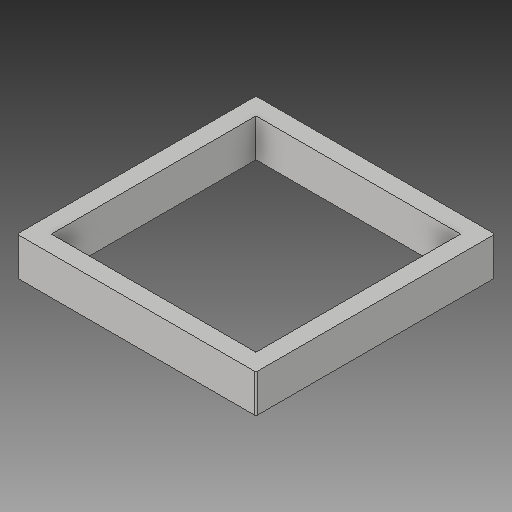
# Autodesk Inventor part: Bumpers
Saved by Autodesk Inventor 2019 (Build 230136000, 136)
## iProperties
Created: 2019-03-14
Part Number: Bumpers
Material: Generic
Document SubType Name: Modeling
Designer: josh
Density: 1 g/cm^3
Appearance: Default
Mass: 29193.8 g
Surface Area: 13341.7 cm^2
Volume: 29193.8 cm^3
Author: josh
Autodesk Inventor part; units mm, degrees
ref_plane "YZ Plane" through (0, 0, 0) normal (1, 0, 0) x (0, 1, 0)
ref_plane "XZ Plane" through (0, 0, 0) normal (0, 1, 0) x (-1, 0, 0)
ref_plane "XY Plane" through (0, 0, 0) normal (0, 0, 1) x (1, 0, 0)
sketch "Sketch5" plane through (0, 0, 0) normal (0, 1, 0) x (-1, 0, 0)
  line L0 (0, 0) -> (755.65, 0)
  line L1 (755.65, 0) -> (755.65, -755.65)
  line L2 (755.65, -755.65) -> (0, -755.65)
  line L3 (0, -755.65) -> (0, 0)
  line L4 (819.15, -812.8) -> (819.15, 57.15)
  line L5 (812.8, 63.5) -> (-57.15, 63.5)
  line L6 (-63.5, 57.15) -> (-63.5, -812.8)
  line L7 (-57.15, -819.15) -> (812.8, -819.15)
  arc A0 (819.15, 57.15) -> (812.8, 63.5) centre (812.8, 57.15) ccw
  arc A1 (812.8, -819.15) -> (819.15, -812.8) centre (812.8, -812.8) ccw
  arc A2 (-63.5, -812.8) -> (-57.15, -819.15) centre (-57.15, -812.8) ccw
  arc A3 (-57.15, 63.5) -> (-63.5, 57.15) centre (-57.15, 57.15) ccw
  dimension "d13" = 755.65
  dimension "d14" = 755.65
  dimension "d15" = 63.5
  dimension "d16" = 6.35
  constraints: 16 end point, 8 point on circle, 8 tangent, 4 centre point, 4 parallel, 3 equal radius, 2 perpendicular, 1 horizontal, 3 other
  measures "d13" distance of L1.end L2.end
  measures "d14" distance of L0.end L1.end
  measures "d15" distance between parallel lines of L1 L4
  measures "d16" radius of A0
extrude "Extrusion2" add sketch "Sketch5" along normal blind 140.335
body "Solid2"
